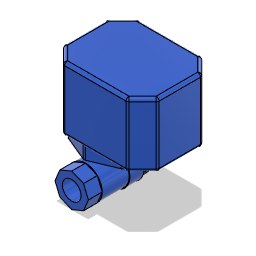
Ball+Valve+(Marine+Mockup) (Autodesk Fusion 360 design; units mm, degrees)
Autodesk Fusion 360 part; units mm, degrees
note: some values were not read from the file. Chosen so that the rebuilt part matches the saved one: which face or edge a step refers to; which pieces of a blend or face edit are solid. Set by a fixed rule: which sketch regions a step uses.
sketch "Sketch2" plane through (0, 0, 0) normal (0, 0, 1) x (1, 0, 0)
  line L0 (20, 0) -> (2.5, 0)
  circle A0 centre (0, 0) radius 6.5
  line L1 (-10.129, -5.2728) -> (-3.4338, -10.8907)
  line L2 (-3.4338, -10.8907) -> (5.2728, -10.129)
  line L3 (5.2728, -10.129) -> (10.8907, -3.4338)
  line L4 (10.8907, -3.4338) -> (10.129, 5.2728)
  line L5 (10.129, 5.2728) -> (3.4338, 10.8907)
  line L6 (3.4338, 10.8907) -> (-5.2728, 10.129)
  line L7 (-5.2728, 10.129) -> (-10.8907, 3.4338)
  line L8 (-10.8907, 3.4338) -> (-10.129, -5.2728)
  dimension "d5" = 13
  dimension "d57" = 10.55
  dimension "d58" = 85
  constraint coincident A0.centre origin
  measures "d5" diameter of A0
  measures "d57" distance of A0.centre L8
  measures "d58" angle of L0 L4
extrude "Extrude1" add sketch "Sketch2" along normal blind 8 makes body 1
sketch "Sketch3" plane through (0, 0, 8) normal (0, 0, 1) x (1, 0, 0)
  circle A0 centre (0, 0) radius 6.5
  circle A1 centre (0, 0) radius 12.125
  line L0 (-10.8907, 3.4338) -> (-10.129, -5.2728)
  line L1 (-10.129, -5.2728) -> (-3.4338, -10.8907)
  line L2 (-3.4338, -10.8907) -> (5.2728, -10.129)
  line L3 (5.2728, -10.129) -> (10.8907, -3.4338)
  line L4 (10.8907, -3.4338) -> (10.129, 5.2728)
  line L5 (10.129, 5.2728) -> (3.4338, 10.8907)
  line L6 (3.4338, 10.8907) -> (-5.2728, 10.129)
  line L7 (-5.2728, 10.129) -> (-10.8907, 3.4338)
  dimension "d6" = 24.25
  constraint coincident A0.centre A1.centre
  measures "d6" diameter of A1
extrude "Extrude2" add sketch "Sketch3" along normal blind 9.9 contours A1 | L0 L1 L2 L3 L4 L5 L6 L7 bodies 1
sketch "Sketch4" plane through (0, 0, 17.9) normal (0, 0, 1) x (1, 0, 0)
  circle A0 centre (0, 0) radius 6.5
  circle A1 centre (0, 0) radius 12.125
  circle A2 centre (0, 0) radius 11.6
  dimension "d9" = 23.2
  constraint concentric A0 A2
  measures "d9" diameter of A2
extrude "Extrude3" add sketch "Sketch4" along normal blind 18.7 contours A2 bodies 1
sketch "Sketch5" plane through (0, 0, 36.6) normal (0, 0, 1) x (1, 0, 0)
  circle A0 centre (0, 0) radius 6.5
  circle A1 centre (0, 0) radius 11.6
  line L0 (-11.6, 0) -> (11.6, 0) construction
  line L1 (8.2024, 8.2024) -> (0, 11.6)
  line L2 (0, 11.6) -> (-8.2024, 8.2024)
  line L3 (-8.2024, 8.2024) -> (-11.6, 0)
  line L4 (-11.6, 0) -> (-8.2024, -8.2024)
  line L5 (-8.2024, -8.2024) -> (0, -11.6)
  line L6 (0, -11.6) -> (8.2024, -8.2024)
  line L7 (8.2024, -8.2024) -> (11.6, 0)
  line L8 (11.6, 0) -> (8.2024, 8.2024)
  constraint coincident A1 L0.start
  constraint coincident A1 L0.end
  constraint horizontal L0
  constraint coincident A0.centre L0
  constraint coincident A0.centre A1.centre
  constraint coincident A1 L1.start
  constraint coincident L0.end L7.end
extrude "Extrude4" add sketch "Sketch5" along normal blind 9.6 contours L1 L2 L3 L4 L5 L6 L7 L8 bodies 1
ref_plane "WorkPlane1" through (0, 12.125, 13.4791) normal (0, 1, 0) x (1, 0, 0)
sketch "Sketch6" plane through (0, 12.125, 13.4791) normal (0, 1, 0) x (1, 0, 0)
  line L0 (11.6, -4.4209) -> (-11.6, -4.4209)
  line L1 (-12.125, -4.4209) -> (12.125, -4.4209)
  line L2 (-12.125, 5.4791) -> (12.125, 5.4791)
  line L3 (0, -23.1209) -> (0, 5.4791) construction
  line L4 (0, -8.8209) -> (10, -8.8209) construction
  line L5 (0, -24.3209) -> (19.5, -16.1959)
  line L6 (19.5, -16.1959) -> (19.5, -8.8209)
  line L7 (0, -24.3209) -> (-19.5, -16.1959)
  line L8 (-19.5, -16.1959) -> (-19.5, -8.8209)
  line L9 (19.5, -1.4459) -> (19.5, -8.8209)
  line L10 (0, 6.6791) -> (19.5, -1.4459)
  line L11 (0, 6.6791) -> (-19.5, -1.4459)
  line L12 (-19.5, -1.4459) -> (-19.5, -8.8209)
  line L13 (-6.364, -7.4067) -> (-1.4142, -2.4569)
  line L14 (1.4142, -2.4569) -> (6.364, -7.4067)
  line L15 (6.364, -10.2351) -> (1.4142, -15.1849)
  line L16 (-1.4142, -15.1849) -> (-6.364, -10.2351)
  arc A0 (-6.364, -7.4067) -> (-6.364, -10.2351) centre (-4.9497, -8.8209) ccw
  arc A1 (6.364, -10.2351) -> (6.364, -7.4067) centre (4.9497, -8.8209) ccw
  arc A2 (1.4142, -2.4569) -> (-1.4142, -2.4569) centre (0, -3.8711) ccw
  arc A3 (-1.4142, -15.1849) -> (1.4142, -15.1849) centre (0, -13.7706) ccw
  line L17 (-11.6, -23.1209) -> (-8.2024, -23.1209)
  line L18 (0, -23.1209) -> (8.2024, -23.1209)
  line L19 (8.2024, -23.1209) -> (11.6, -23.1209)
  line L20 (8.2024, -23.1209) -> (11.6, -23.1209)
  line L21 (0, -23.1209) -> (8.2024, -23.1209)
  line L22 (-8.2024, -23.1209) -> (0, -23.1209)
  line L23 (-11.6, -23.1209) -> (-8.2024, -23.1209)
  line L24 (-8.2024, -23.1209) -> (0, -23.1209)
  dimension "d15" = 10
  dimension "d16" = 39
  dimension "d17" = 14.75
  dimension "d18" = 2
  dimension "d19" = 31
  dimension "d20" = 11
  constraint midpoint L3 L4.start
  constraint perpendicular L3 L4
  constraint coincident L3 L5.start
  constraint parallel L3 L6
  constraint symmetric L3 L5.start L7.start
  constraint symmetric L3 L5.end L7.end
  constraint symmetric L3 L6.end L8.end
  constraint symmetric L4 L5.start L10.start
  constraint symmetric L4 L5.end L9.start
  constraint symmetric L4 L6.end L9.end
  constraint symmetric L4 L7.end L11.end
  constraint symmetric L4 L8.end L12.end
  constraint coincident L6.end L9.end
  constraint perpendicular L13 L14
  constraint parallel L13 L15
  constraint parallel L14 L16
  constraint tangent L13 A0
  constraint tangent L16 A0
  constraint tangent L14 A1
  constraint tangent L15 A1
  constraint equal A0 A1
  constraint tangent L13 A2
  constraint tangent L14 A2
  constraint equal A0 A2
  constraint tangent L15 A3
  constraint tangent L16 A3
  constraint equal A0 A3
  constraint coincident L4 A1.centre
  constraint coincident L3 A3.centre
  constraint coincident L3 A2.centre
  constraint coincident L4 A0.centre
  measures "d15" distance of L4.start L4.end
  measures "d16" distance of L6 L8
  measures "d17" distance of L5.end L9.start
  measures "d18" radius of A0
  measures "d19" distance of L5.start L10.start
  measures "d20" distance of L13 L15
extrude "Extrude5" add sketch "Sketch6" along normal up to surface and the other way blind -2 contours L0 L1 L13 L14 L15 L16 A0 A1 A3 | L0 L1 L13 L14 A2 end surface at (-10.0459, 5.8, 24.1333) on bodies 1 bodies 1
sketch "Sketch7" plane through (0, 14.125, 0) normal (0, 1, 0) x (-1, 0, 0)
  arc A0 (6.364, 20.8858) -> (6.364, 23.7142) centre (4.9497, 22.3) ccw
  line L0 (6.364, 23.7142) -> (1.4142, 28.664)
  arc A1 (1.4142, 28.664) -> (-1.4142, 28.664) centre (0, 27.2497) ccw
  line L1 (-1.4142, 28.664) -> (-6.364, 23.7142)
  arc A2 (-6.364, 23.7142) -> (-6.364, 20.8858) centre (-4.9497, 22.3) ccw
  line L2 (-6.364, 20.8858) -> (-1.4142, 15.936)
  arc A3 (-1.4142, 15.936) -> (1.4142, 15.936) centre (0, 17.3503) ccw
  line L3 (1.4142, 15.936) -> (6.364, 20.8858)
  line L4 (19.5, 14.925) -> (19.5, 22.3)
  line L5 (19.5, 29.675) -> (19.5, 22.3)
  line L6 (0, 37.8) -> (19.5, 29.675)
  line L7 (0, 37.8) -> (-19.5, 29.675)
  line L8 (-19.5, 29.675) -> (-19.5, 22.3)
  line L9 (-19.5, 14.925) -> (-19.5, 22.3)
  line L10 (0, 6.8) -> (-19.5, 14.925)
  line L11 (0, 6.8) -> (19.5, 14.925)
extrude "Extrude6" add sketch "Sketch7" along normal blind 9.5 separate body contours A0 L0 A1 L1 A2 L2 A3 L3 | L4 L5 L6 L7 L8 L9 L10 L11 makes body 2
sketch "Sketch8" plane through (0, 23.625, 0) normal (0, 1, 0) x (-1, 0, 0)
  line L0 (-19.5, 14.925) -> (0, 6.8)
  line L1 (0, 6.8) -> (19.5, 14.925)
  line L2 (19.5, 14.925) -> (19.5, 29.675)
  line L3 (19.5, 29.675) -> (0, 37.8)
  line L4 (0, 37.8) -> (-19.5, 29.675)
  line L5 (-19.5, 29.675) -> (-19.5, 14.925)
  line L6 (22.7, 39.8) -> (-42.8, 39.8)
  line L7 (-42.8, 39.8) -> (-42.8, -11.9)
  line L8 (-42.8, -11.9) -> (22.7, -11.9)
  line L9 (22.7, -11.9) -> (22.7, 39.8)
  line L10 (22.7, -1.2934) -> (12.0934, -11.9)
  line L11 (-32.1934, -11.9) -> (-42.8, -1.2934)
  line L12 (-42.8, 29.1934) -> (-32.1934, 39.8)
  line L13 (22.7, 29.1934) -> (12.0934, 39.8)
  dimension "d27" = 65.5
  dimension "d28" = 51.7
  dimension "d29" = 2
  dimension "d30" = 3.2
  dimension "d32" = 45
  dimension "d33" = 45
  dimension "d34" = 15
  dimension "d35" = 15
  dimension "d36" = 15
  dimension "d37" = 15
  dimension "d38" = 45
  constraint horizontal L6
  constraint vertical L7
  constraint horizontal L8
  constraint vertical L9
  constraint coincident L9 L10.start
  constraint coincident L8 L10.end
  constraint coincident L8 L11.start
  constraint coincident L7 L11.end
  constraint coincident L7 L12.start
  constraint coincident L6 L12.end
  constraint coincident L9 L13.start
  constraint coincident L6 L13.end
  constraint perpendicular L12 L13
  measures "d27" distance of L7.end L8.end
  measures "d28" distance of L6.end L7.end
  measures "d29" distance of L3.end L6
  measures "d30" distance of L2 L9
  measures "d32" angle of L6 L13
  measures "d33" angle of L8 L11
  measures "d34" distance of L11.start L11.end
  measures "d35" distance of L12.start L12.end
  measures "d36" distance of L13.start L13.end
  measures "d37" distance of L10.start L10.end
  measures "d38" angle of L8 L10
extrude "Extrude7" add sketch "Sketch8" along normal blind 44.5 contours L0 L1 L2 L3 L4 L5 | L6 L7 L8 L9 L10 L11 L12 L13 bodies 2
fillet "Fillet1" radius 2 9 faces at (17.4311, 68.125, 5.3333) (-22.7, 53.2917, 8.8689) (-19.1645, 38.4583, -4.8289) (17.4311, 38.4583, -11.9) (35.7289, 38.4583, -8.3645) (42.8, 53.2917, 19.0311) (39.2645, 38.4583, 32.7289) (17.4311, 53.2917, 39.8) (-19.1645, 38.4583, 32.7289) on bodies 2
fillet "Fillet2" radius 2 6 edges at (-19.5, 18.8758, 29.675) (0, 18.875, 37.8) (-19.5, 18.875, 14.925) (19.5, 18.875, 29.675) (19.5, 18.875, 14.925) (0, 18.875, 6.8) on bodies 2
combine "Combine1" operation add target body 1 tool bodies 2
sketch "Sketch9" plane through (0, 0, 0) normal (0, 0, -1) x (-1, 0, 0)
  circle A0 centre (0, 0) radius 6.5
  circle A1 centre (0, 0) radius 8
  circle A2 centre (0, 0) radius 6.7
  line L0 (0.5489, 7.9811) -> (-6.6374, 4.4659)
  line L1 (-6.6374, 4.4659) -> (-7.1863, -3.5152)
  line L2 (-7.1863, -3.5152) -> (-0.5489, -7.9811)
  line L3 (-0.5489, -7.9811) -> (6.6374, -4.4659)
  line L4 (6.6374, -4.4659) -> (7.1863, 3.5152)
  line L5 (7.1863, 3.5152) -> (0.5489, 7.9811)
  line L6 (10.129, -5.2728) -> (10.8907, 3.4338)
  line L7 (10.8907, 3.4338) -> (5.2728, 10.129)
  line L8 (5.2728, 10.129) -> (-3.4338, 10.8907)
  line L9 (-3.4338, 10.8907) -> (-10.129, 5.2728)
  line L10 (-10.129, 5.2728) -> (-10.8907, -3.4338)
  line L11 (-10.8907, -3.4338) -> (-5.2728, -10.129)
  line L12 (-5.2728, -10.129) -> (3.4338, -10.8907)
  line L13 (3.4338, -10.8907) -> (10.129, -5.2728)
  dimension "d45" = 13.4
  dimension "d46" = 16
  constraint concentric A0 A1
  constraint concentric A1 A2
  constraint coincident A1 L0.start
  constraint coincident A0.centre A1.centre
  measures "d45" diameter of A2
  measures "d46" diameter of A1
